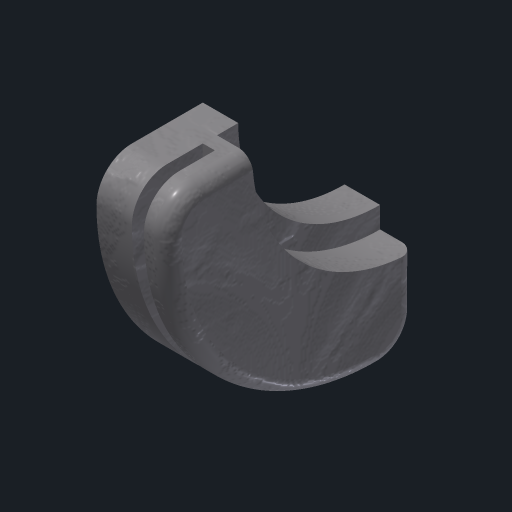
# Autodesk Inventor part: ESQUINERO_PUERTAS
Saved by Autodesk Inventor 2024.3 (Build 283343000, 343)
## iProperties
Created: 2024-07-05
Part Number: ESQUINERO_PUERTAS
Material: Steel, Mild, Welded
Document SubType Name: Modeling
Designer: Niler
Density: 7.85 g/cm^3
Appearance: Weld - Steel Mild
Author: Niler
Autodesk Inventor part; units mm, degrees
ref_plane "YZ Plane" through (0, 0, 0) normal (1, 0, 0) x (0, 1, 0)
ref_plane "XZ Plane" through (0, 0, 0) normal (0, 1, 0) x (-1, 0, 0)
ref_plane "XY Plane" through (0, 0, 0) normal (0, 0, 1) x (1, 0, 0)
sketch "Sketch1" plane through (0, 0, 0) normal (1, 0, 0) x (0, 1, 0)
  line L0 (0, 0) -> (50, 0)
  line L1 (50, 0) -> (50, -50)
  line L2 (50, -50) -> (0, -50)
  line L3 (0, -50) -> (0, 0)
  circle A0 centre (25, -25) radius 25
  line L4 (25, 0) -> (25, 10)
  line L5 (25, 10) -> (-10, 10)
  line L6 (-10, 10) -> (-10, -25)
  line L7 (-10, -25) -> (0, -25)
  line L8 (25, 0) -> (25, -25)
  line L9 (25, -25) -> (0, -25)
  circle A1 centre (25, -25) radius 20
  circle A2 centre (25, -25) radius 23
  point P0 (50, -25)
  point P1 (25, -50)
  point P2 (2, -25)
  point P3 (25, -2)
  point P4 (5, -25)
  point P5 (25, -5)
  dimension "d0" = 50
  dimension "d1" = 5
  dimension "d2" = 35
  dimension "d3" = 2
  constraints: 20 end point, 6 perpendicular, 4 midpoint, 3 centre point, 2 parallel, 2 point on circle, 2 tangent, 1 collinear, 1 horizontal, 1 horizontal alignment, 1 vertical, 1 vertical alignment
  measures "d0" distance of L0.end L1.end
  measures "d1" radial gap between concentric circles of A0 A1
  measures "d2" distance of L4.end L5.end
  measures "d3" radial gap between concentric circles of A0 A2
extrude "Extrusion1" add sketch "Sketch1" along normal blind 5 contours L3 L7 L6 L5 L4 L0 | L0 A0 L3 | L8 A2 L9 A0 picked at (1.8931, -17.824)
extrude "Extrusion2" add sketch "Sketch1" against normal blind 5 contours L3 L7 L6 L5 L4 L0 | L0 A0 L3 | L8 A2 L9 A0 | L8 A1 L9 A2 picked at (1.8931, -17.824) picked at (4.6117, -17.075)
extrude "Extrusion3" cut sketch "Sketch1" along normal blind 1.7 contours L3 L7 L6 L5 L4 L0
fillet "Fillet1" radius 30 2 edges at (3.35, -10, 10) (-2.5, -10, 10)
fillet "Fillet2" radius 5 4 edges at (3.35, 25, 10) (-2.5, 25, 10) (3.35, -10, -25) (-2.5, -10, -25)
fillet "Fillet3" radius 2 7 edges at (5, -10, -20.0001) (5, -1.2132, 1.2132) (5, 20, 10) (5, -8.5356, -23.5356) (5, -1.5, -25) (5, 23.5356, 8.5356) (5, 25, 1.5)
body "Solid1"
